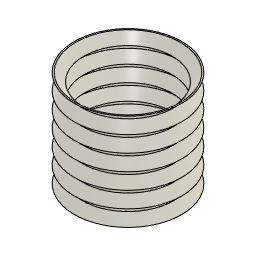
TestBellows v1 (Autodesk Fusion 360 design; units mm, degrees)
Autodesk Fusion 360 part; units mm, degrees
sketch "Sketch1" plane through (0, 0, 0) normal (0, 1, 0) x (1, 0, 0)
  line L0 (32.5, 0) -> (27.5, -5)
  line L1 (27.5, -5) -> (32.5, -10)
  line L2 (33.4, 0) -> (28.4, -5)
  line L3 (28.4, -5) -> (33.4, -10)
  line L4 (32.5, 0) -> (33.4, 0)
  line L5 (33.4, -10) -> (32.5, -10)
  line L6 (32.5, 0) -> (0, 0) construction
  point P0 (30, -2.5)
  dimension "d1" = 0.9
  dimension "d2" = 10
  dimension "d11" = 30
  dimension "d12" = 32.5
  constraint perpendicular L0 L1
  constraint perpendicular L1 L2
  constraint perpendicular L2 L3
  constraint horizontal L0.end L2.end
  constraint horizontal L5
  constraint horizontal L4
  constraint coincident L6.end origin
  constraint horizontal L6
  constraint equal L2 L3
  constraint vertical L2.start L3.end
  constraint midpoint L0 P0
  measures "d1" distance of L0.start L2.start
  measures "d2" distance of L2.start L3.end
  measures "d11" horizontal distance of L6.end P0
  measures "d12" distance of L0.start L6.end
revolve "Revolve1" add sketch "Sketch1" angle 360 about axis through (0, 0, 1.75) along (0, 0, 1) makes body 1
pattern_linear "R-Pattern1" count 6 spacing 10 along (0, 0, 1) of bodies 1 makes body 2 at (31.5756, -3.1596, 18.3333) makes body 3 at (31.5756, -3.1596, 28.3333) makes body 4 at (31.5756, -3.1596, 38.3333) makes body 5 at (31.5756, -3.1596, 48.3333) makes body 6 at (31.5756, -3.1596, 58.3333)
combine "Combine1" operation add target body 1 tool bodies 2 4 5 6 3
